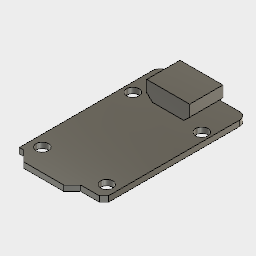
1501 Trinket 5V (Autodesk Fusion 360 design; units mm, degrees)
Autodesk Fusion 360 part; units mm, degrees
sketch "remake" plane through (0, 0, 0) normal (0, 0, 1) x (1, 0, 0)
  line L0 (-7.62, -13.32) -> (7.62, -13.32)
  line L1 (7.62, -13.32) -> (7.62, 13.32)
  line L2 (7.62, 13.32) -> (-7.62, 13.32)
  line L3 (-7.62, 13.32) -> (-7.62, -13.32)
  line L4 (-7.62, -13.32) -> (7.62, 13.32) construction
  line L5 (7.62, -13.32) -> (-7.62, 13.32) construction
  circle A0 centre (-6.1, 6.3) radius 1.1
  line L6 (0, 13.32) -> (0, 0) construction
  circle A1 centre (6.1, 6.3) radius 1.1
  circle A2 centre (-5.34, -10.2) radius 1.09
  circle A3 centre (5.34, -10.2) radius 1.09
  dimension "d3" = 26.64
  dimension "d4" = 15.24
  dimension "d5" = 2.2
  dimension "d6" = 6.3
  dimension "d7" = 6.1
  dimension "d13" = 2.18
  dimension "d14" = 5.34
  dimension "d15" = 16.5
  measures "d3" distance of L0.end L1.end
  measures "d4" distance of L1.end L2.end
  measures "d5" diameter of A0
  measures "d6" distance of L6.end A0.centre
  measures "d7" distance of L6.end A0.centre
  measures "d13" diameter of A2
  measures "d14" distance of L6.end A2.centre
  measures "d15" distance of A0.centre A2.centre
extrude "Extrude2" add sketch "remake" along normal blind 1 makes body 1
sketch "remake tester" plane through (0, 0, 0) normal (0, 0, -1) x (1, 0, 0)
  circle A0 centre (-5.34, 10.2) radius 1.09
  circle A1 centre (6.1, -6.3) radius 1.1
  circle A2 centre (5.34, 10.2) radius 1.09
  circle A3 centre (-6.1, -6.3) radius 1.1
  line L0 (-7.62, 13.32) -> (-7.62, -13.32) construction
  line L1 (-7.62, -13.32) -> (7.62, -13.32) construction
  line L2 (7.62, -13.32) -> (7.62, 13.32) construction
  line L3 (7.62, 13.32) -> (-7.62, 13.32) construction
  circle A4 centre (-5.34, 10.2) radius 2.5
  circle A5 centre (5.34, 10.2) radius 2.5
  circle A6 centre (-6.1, -6.3) radius 2.5
  circle A7 centre (6.1, -6.3) radius 2.5
  line L4 (-9.62, -15.32) -> (9.62, -15.32)
  line L5 (9.62, -15.32) -> (9.62, 15.32)
  line L6 (9.62, 15.32) -> (-9.62, 15.32)
  line L7 (-9.62, 15.32) -> (-9.62, -15.32)
  dimension "d18" = 5
  dimension "d19" = 5
  dimension "d20" = 5
  dimension "d21" = 5
  dimension "d22" = 2
  measures "d18" diameter of A4
  measures "d19" diameter of A5
  measures "d20" diameter of A6
  measures "d21" diameter of A7
extrude "Extrude3" add sketch "remake tester" along normal blind 3 and the other way blind -2 separate body contours A0 | A1 | A2 | A3 | A4 | A5 | A6 | A7 | L4 L5 L6 L7 makes body 2
extrude "Extrude4" add sketch "remake tester" along normal blind 2 contours A0 | A1 | A2 | A3 | A4 | A5 | A6 | A7 bodies 2
extrude "Extrude5" add sketch "remake tester" against normal blind 2 contours A0 | A1 | A2 | A3 bodies 2
sketch "trinket import" plane through (0, 0, 0) normal (0, 0, 1) x (1, 0, 0)
  line L0 (2.7, 13.8) -> (2.5, 13.5)
  line L1 (2.5, 13.5) -> (-2.6, 13.5)
  line L2 (-2.6, 13.5) -> (-2.8, 13.8)
  line L3 (-2.8, 13.8) -> (-6.4, 13.8)
  spline S0 degree 3 poles (-6.4, 13.8) (-7.1, 13.8) (-7.7, 13.2) (-7.7, 12.5) knots 0 0 0 0 1 1 1 1
  line L4 (-7.7, 12.5) -> (-7.7, -11.1)
  line L5 (-7.7, -11.1) -> (-6.9, -11.1)
  line L6 (-6.9, -11.1) -> (-5.1, -12.9)
  line L7 (-5.1, -12.9) -> (2, -12.9)
  line L8 (2, -12.9) -> (3.5, -11.4)
  line L9 (3.5, -11.4) -> (6.8, -11.4)
  line L10 (6.8, -11.4) -> (7.6, -10.6)
  line L11 (7.6, -10.6) -> (7.6, 12.6)
  spline S1 degree 3 poles (7.6, 12.6) (7.6, 13.3) (7, 13.9) (6.3, 13.9) knots 0 0 0 0 1 1 1 1
  line L12 (6.3, 13.9) -> (2.7, 13.9)
  line L13 (2.7, 13.9) -> (2.7, 13.8)
  circle A0 centre (-6.1, 7.4) radius 1.105
  circle A1 centre (6.1, 7.4) radius 1.105
  circle A2 centre (-5.7, -9) radius 1.09
  circle A3 centre (5.7, -9) radius 1.09
  dimension "d30" = 2.21
  dimension "d31" = 2.21
  dimension "d32" = 2.18
  dimension "d33" = 2.18
  measures "d30" diameter of A0
  measures "d31" diameter of A1
  measures "d32" diameter of A2
  measures "d33" diameter of A3
extrude "Extrude6" add sketch "trinket import" along normal blind 1 separate body makes body 3
sketch "trinket tester" plane through (0, 0, 0) normal (0, 0, -1) x (1, 0, 0)
  circle A0 centre (-6.1, -7.4) radius 1.105
  circle A1 centre (5.7, 9) radius 1.09
  circle A2 centre (6.1, -7.4) radius 1.105
  circle A3 centre (-5.7, 9) radius 1.09
  line L0 (2.7, -13.8) -> (2.7, -13.9)
  line L1 (2.7, -13.9) -> (6.3, -13.9)
  spline S0 degree 3 poles (7.6, -12.6) (7.6, -13.3) (7, -13.9) (6.3, -13.9) knots 0 0 0 0 1 1 1 1
  line L2 (7.6, -12.6) -> (7.6, 10.6) construction
  line L3 (7.6, 10.6) -> (6.8, 11.4)
  line L4 (6.8, 11.4) -> (3.5, 11.4) construction
  line L5 (3.5, 11.4) -> (2, 12.9)
  line L6 (2, 12.9) -> (-5.1, 12.9)
  line L7 (-5.1, 12.9) -> (-6.9, 11.1) construction
  line L8 (-6.9, 11.1) -> (-7.7, 11.1) construction
  line L9 (-7.7, 11.1) -> (-7.7, -12.5) construction
  spline S1 degree 3 poles (-6.4, -13.8) (-7.1, -13.8) (-7.7, -13.2) (-7.7, -12.5) knots 0 0 0 0 1 1 1 1
  line L10 (-6.4, -13.8) -> (-2.8, -13.8)
  line L11 (-2.8, -13.8) -> (-2.6, -13.5)
  line L12 (-2.6, -13.5) -> (2.5, -13.5)
  line L13 (2.5, -13.5) -> (2.7, -13.8)
  circle A4 centre (-5.7, 9) radius 3
  circle A5 centre (5.7, 9) radius 3
  circle A6 centre (-6.1, -7.4) radius 3
  circle A7 centre (6.1, -7.4) radius 3
  line L14 (-10, -13.5) -> (10, -13.5)
  line L15 (10, -13.5) -> (10, 13.5)
  line L16 (10, 13.5) -> (-10, 13.5)
  line L17 (-10, 13.5) -> (-10, -13.5)
  line L18 (-10, -13.5) -> (10, 13.5) construction
  line L19 (10, -13.5) -> (-10, 13.5) construction
  dimension "d36" = 6
  dimension "d37" = 6
  dimension "d38" = 6
  dimension "d39" = 6
  dimension "d40" = 20
  dimension "d41" = 27
  measures "d36" diameter of A4
  measures "d37" diameter of A5
  measures "d38" diameter of A6
  measures "d39" diameter of A7
  measures "d40" distance of L15.end L16.end
  measures "d41" distance of L14.end L15.end
extrude "Extrude7" add sketch "trinket tester" along normal blind 4 and the other way blind -3 separate body contours A0 | A1 | A2 | A3 | L12 L14 L15 L16 L17 | A4 | A5 | A6 | A7 makes body 4
extrude "Extrude8" add sketch "trinket tester" along normal up to surface (3 mm away) contours A0 | A1 | A2 | A3 | A4 | A5 | A6 | A7 bodies 4
extrude "Extrude9" cut sketch "trinket tester" along normal blind 10 contours A0 | A1 | A2 | A3 bodies 4
chamfer "Chamfer1" distance 1 angle 45 4 edges at (-6.7162, -9.3942, -4) (4.6838, -9.3942, -4) (-7.1302, 7.0004, -4) (5.0698, 7.0004, -4) on bodies 4
sketch "Sketch12" plane through (0, 13.5, 0) normal (0, 1, 0) x (-1, 0, 0)
  line L0 (-2.5, 0) -> (2.6, 0)
  line L1 (2.6, 0) -> (2.6, 1)
  line L2 (2.6, 1) -> (-2.5, 1)
  line L3 (-2.5, 1) -> (-2.5, 0)
  line L4 (0.05, 1) -> (0.05, 3.5) construction
  line L5 (3.85, 1) -> (-3.75, 1)
  line L6 (-3.75, 1) -> (-3.75, 4)
  line L7 (-3.75, 4) -> (3.85, 4)
  line L8 (3.85, 4) -> (3.85, 1)
  line L9 (3.85, 1) -> (-3.75, 4) construction
  line L10 (-3.75, 1) -> (3.85, 4) construction
  point P0 (0.05, 2.5)
  dimension "d49" = 7.6
  dimension "d50" = 3
  measures "d49" distance of L6.end L7.end
  measures "d50" distance of L5.end L6.end
extrude "Extrude10" add sketch "Sketch12" against normal blind 5.9 separate body contours L2 L5 L6 L7 L8 makes body 5
chamfer "Chamfer2" distance 1 angle 45 2 edges at (3.75, 10.55, 1) (-3.85, 10.55, 1) on bodies 5
hidden bodies 1 2 4
named bodies: "trinket PCB", "trinket tester", "MicroUSB"
